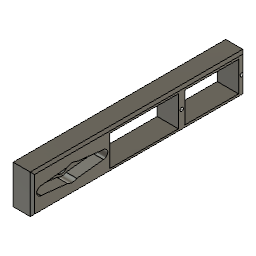
Arm00 (Autodesk Fusion 360 design; units mm, degrees)
part number: 2026-06-04-10-46-39-253
Autodesk Fusion 360 part; units mm, degrees
sketch "Sketch1" plane through (0, 0, 0) normal (0, 0, 1) x (1, 0, 0)
  line L0 (5, -50) -> (-5, -50)
  line L1 (-5, -50) -> (-5, 50)
  line L2 (-5, 50) -> (5, 50)
  line L3 (5, 50) -> (5, -50)
  line L4 (5, -50) -> (-5, 50) construction
  line L5 (-5, -50) -> (5, 50) construction
  dimension "d1" = 10
  dimension "d2" = 100
  constraint horizontal L0
  constraint perpendicular L0 L1
  constraint parallel L0 L2
  constraint parallel L1 L3
  constraint coincident L4 origin
  constraint coincident L5 origin
  measures "d1" distance of L1.end L2.end
  measures "d2" distance of L0.end L1.end
extrude "Extrude1" add sketch "Sketch1" along normal blind 20
sketch "Sketch2" plane through (5, 0, 0) normal (1, 0, 0) x (0, 1, 0)
  line L0 (-50, 0) -> (50, 0)
  line L1 (50, 0) -> (50, 20)
  line L2 (50, 20) -> (-50, 20)
  line L3 (-50, 20) -> (-50, 0)
  line L4 (21, 17) -> (46, 17)
  line L5 (46, 17) -> (46, 3)
  line L6 (46, 3) -> (21, 3)
  line L7 (21, 3) -> (21, 17)
  dimension "d15" = 25
  dimension "d16" = 14
  dimension "d17" = 4
  dimension "d18" = 3
  constraint horizontal L4
  constraint vertical L5
  constraint horizontal L6
  constraint vertical L7
  measures "d15" distance of L4.start L4.end
  measures "d16" distance of L4.start L6.end
  measures "d17" distance of L1 L5
  measures "d18" distance of L2 L4.end
extrude "Extrude2" cut sketch "Sketch2" against normal blind 10 contours L4 L5 L6 L7
sketch "NozzleSketch" plane through (5, 0, 0) normal (1, 0, 0) x (0, 1, 0)
  arc A0 (-46, 12) -> (-46, 8) centre (-46, 10) ccw
  line L0 (-46, 8) -> (-46, 12)
  arc A1 (-16.9496, 8) -> (-16.9496, 12) centre (-16.9496, 10) ccw
  line L1 (-16.9496, 12) -> (-16.9496, 8)
  circle A2 centre (-31.3885, 10) radius 4
  line L2 (-29.2976, 6.59) -> (-16.9496, 8)
  line L3 (-16.9496, 12) -> (-29.2976, 13.41)
  line L4 (-33.6516, 13.2982) -> (-46, 12)
  line L5 (-46, 8) -> (-33.6516, 6.7018)
  line L6 (-50, 0) -> (-50, 20)
  line L7 (-48, 10) -> (-50, 10) construction
  point P0 (-48, 10)
  point P1 (-14.9496, 10)
  dimension "d89" = 8
  dimension "d90" = 2
  dimension "d91" = 2
  dimension "d92" = 12.3484
  dimension "d93" = 12.3484
  dimension "d94" = 12.348
  dimension "d95" = 12.348
  dimension "d96" = 2
  constraint coincident A0.centre L0
  constraint coincident A1.centre L1
  constraint midpoint P0 A0
  constraint midpoint P1 A1
  constraint horizontal P0 A0.centre
  constraint horizontal A0.centre A2.centre
  constraint horizontal A1.centre A2.centre
  constraint horizontal P1 A1.centre
  constraint coincident A2 L3.end
  constraint coincident A2 L2.start
  constraint coincident A2 L4.start
  constraint coincident A2 L5.end
  constraint coincident P0 L7.start
  constraint midpoint L6 L7.end
  constraint horizontal L7
  measures "d89" diameter of A2
  measures "d90" radius of A0
  measures "d91" radius of A1
  measures "d92" horizontal distance of A0.start L4.start
  measures "d93" horizontal distance of A0.end L5.end
  measures "d94" horizontal distance of A1.start L2.start
  measures "d95" horizontal distance of A1.end L3.end
  measures "d96" distance of P0 L6
extrude "Extrude10" cut sketch "NozzleSketch" against normal blind 5
sketch "Sketch5" plane through (5, 0, 0) normal (1, 0, 0) x (0, 1, 0)
  line L0 (46, 17) -> (46, 3)
  line L1 (46, 3) -> (21, 3)
  line L2 (21, 3) -> (21, 17)
  line L3 (21, 17) -> (46, 17)
  line L4 (-50, 0) -> (50, 0)
  line L5 (50, 0) -> (50, 20)
  line L6 (50, 20) -> (-50, 20)
  line L7 (-50, 20) -> (-50, 0)
  line L8 (-29.2976, 13.41) -> (-16.9496, 12)
  arc A0 (-16.9496, 8) -> (-16.9496, 12) centre (-16.9496, 10) ccw
  line L9 (-16.9496, 8) -> (-29.2976, 6.59)
  arc A1 (-46, 12) -> (-46, 8) centre (-46, 10) ccw
  line L10 (-46, 12) -> (-33.6516, 13.2982)
  arc A2 (-29.2976, 13.41) -> (-33.6516, 13.2982) centre (-31.3885, 10) ccw
  arc A3 (-33.6516, 6.7018) -> (-29.2976, 6.59) centre (-31.3885, 10) ccw
  line L11 (-33.6516, 6.7018) -> (-46, 8)
  point P0 (19.5, 10)
  point P1 (47.5, 10)
  dimension "d46" = 1.5
  dimension "d47" = 1.5
  dimension "d48" = 10
  dimension "d49" = 10
  measures "d46" distance of L2 P0
  measures "d47" distance of L0 P1
  measures "d48" distance of L6 P1
  measures "d49" distance of L6 P0
hole "Hole4" at (5, 47.5, 10) at (5, 19.5, 10) direction (-1, 0, 0) diameter 1.623 depth 6 tip angle 118
thread "Thread3" "ISO Metric profile 2.0 M2x0.4 M2x0.4 6H" thread offset 0 thread depth 7.4
sketch "Sketch7" plane through (5, 0, 0) normal (1, 0, 0) x (0, 1, 0)
  circle A0 centre (47.5, 10) radius 0.8115
  circle A1 centre (19.5, 10) radius 0.8115
  line L0 (46, 17) -> (46, 3)
  line L1 (46, 3) -> (21, 3)
  line L2 (21, 3) -> (21, 17)
  line L3 (21, 17) -> (46, 17)
  line L4 (-50, 0) -> (50, 0)
  line L5 (50, 0) -> (50, 20)
  line L6 (50, 20) -> (-50, 20)
  line L7 (-50, 20) -> (-50, 0)
  line L8 (-13.9496, 17.0815) -> (18, 17.0815)
  line L9 (18, 17.0815) -> (18, 2.9185)
  line L10 (18, 2.9185) -> (-13.9496, 2.9185)
  line L11 (-13.9496, 2.9185) -> (-13.9496, 17.0815)
  line L12 (-13.9496, 2.9185) -> (-13.9496, 17.0815) construction
  arc A2 (-33.6516, 6.7018) -> (-29.2976, 6.59) centre (-31.3885, 10) ccw
  line L13 (-33.6516, 6.7018) -> (-46, 8)
  arc A3 (-46, 12) -> (-46, 8) centre (-46, 10) ccw
  line L14 (-46, 12) -> (-33.6516, 13.2982)
  arc A4 (-29.2976, 13.41) -> (-33.6516, 13.2982) centre (-31.3885, 10) ccw
  line L15 (-29.2976, 13.41) -> (-16.9496, 12)
  arc A5 (-16.9496, 8) -> (-16.9496, 12) centre (-16.9496, 10) ccw
  line L16 (-16.9496, 8) -> (-29.2976, 6.59)
  point P0 (-13.9496, 10)
  dimension "d62" = 10
  dimension "d71" = 3
  dimension "d99" = 3
  constraint horizontal L8
  constraint vertical L9
  constraint horizontal L10
  constraint vertical L11
  constraint midpoint L12 P0
  constraint coincident L11 P0
  measures "d62" distance of L4 P0
  measures "d71" distance of L2 L9
  measures "d99" distance of L11 A5.centre
extrude "Extrude5" cut sketch "Sketch7" against normal blind 10 contours L8 L9 L10 L11
extrude "Extrude6" cut 1 faces at (1.6667, -16.6667, 20) along direction (0, 0, -1) blind 1
extrude "Extrude7" cut 1 faces at (1.6667, -16.6667, 0) along direction (0, 0, 1) blind 1
extrude "Extrude8" cut 1 faces at (-1.6667, 50, 13) along direction (0, -1, 0) blind 1
chamfer "Chamfer2" distance 1 angle 45 8 edges at (5, -0.5, 1) (5, -50, 10) (5, -0.5, 19) (5, 49, 10) (-5, -0.5, 19) (-5, -50, 10) (-5, -0.5, 1) (-5, 49, 10)
sketch "Sketch11" plane through (0, 0, 0) normal (1, 0, 0) x (0, 1, 0)
  line L0 (-46, 8) -> (-33.6516, 6.7018)
  arc A0 (-33.6516, 6.7018) -> (-29.2976, 6.59) centre (-31.3885, 10) ccw
  line L1 (-29.2976, 6.59) -> (-16.9496, 8)
  arc A1 (-16.9496, 8) -> (-16.9496, 12) centre (-16.9496, 10) ccw
  line L2 (-16.9496, 12) -> (-29.2976, 13.41)
  arc A2 (-29.2976, 13.41) -> (-33.6516, 13.2982) centre (-31.3885, 10) ccw
  line L3 (-33.6516, 13.2982) -> (-46, 12)
  arc A3 (-46, 12) -> (-46, 8) centre (-46, 10) ccw
  line L4 (-49, 2) -> (-49, 18)
  point P0 (-45.3885, 10)
  point P1 (-17.3885, 10)
  point P2 (-49, 10)
  dimension "d100" = 14
  dimension "d101" = 14
  constraint midpoint P2 L4
  constraint horizontal P0 P2
  constraint horizontal P0 P1
  measures "d100" distance of A0.centre P0
  measures "d101" horizontal distance of A0.centre P1
hole "Hole5" at (0, -17.3885, 10) at (0, -45.3885, 10) direction (-1, 0, 0) diameter 2.076 depth 3 tip angle 118
thread "Thread4" "ISO Metric profile 2.5 M2.5x0.45 M2.5x0.45 6H" thread offset 0 thread depth 7.4
hole "Hole7" at (0, -31.3885, 10) direction (-1, 0, 0) diameter 6 depth 5 tip angle 180
